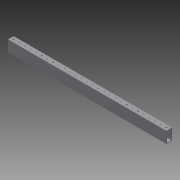
# Autodesk Inventor part: frame_wide
Saved by Autodesk Inventor 2015 SP1 (Build 190203100, 203)
## iProperties
Created: 2014-12-21
Part Number: frame_wide
Material: Generic
Document SubType Name: Modeling
Designer: Jarod
Density: 1 g/cm^3
Appearance: Default
Author: Jarod
Autodesk Inventor part; units mm, degrees
ref_plane "YZ Plane" through (0, 0, 0) normal (1, 0, 0) x (0, 1, 0)
ref_plane "XZ Plane" through (0, 0, 0) normal (0, 1, 0) x (-1, 0, 0)
ref_plane "XY Plane" through (0, 0, 0) normal (0, 0, 1) x (1, 0, 0)
sketch "Sketch1" plane through (0, 0, 0) normal (1, 0, 0) x (0, 1, 0)
  line L0 (0, 0) -> (50.8, 0)
  line L1 (50.8, 0) -> (50.8, -25.4)
  line L2 (50.8, -25.4) -> (0, -25.4)
  line L3 (0, -25.4) -> (0, 0)
  line L4 (2.54, -2.54) -> (48.26, -2.54)
  line L5 (48.26, -2.54) -> (48.26, -22.86)
  line L6 (48.26, -22.86) -> (2.54, -22.86)
  line L7 (2.54, -22.86) -> (2.54, -2.54)
  dimension "d0" = 50.8
  dimension "d1" = 25.4
  dimension "d2" = 45.72
  dimension "d3" = 20.32
  dimension "d4" = 2.54
  dimension "d5" = 2.54
  constraints: 16 end point, 4 parallel, 2 horizontal, 2 perpendicular
  measures "d0" distance of L1.end L2.end
  measures "d1" distance of L0.end L1.end
  measures "d2" distance of L5.end L6.end
  measures "d3" distance of L4.end L5.end
  measures "d4" distance between parallel lines of L4 L0
  measures "d5" distance between parallel lines of L3 L7
extrude "Extrusion1" add sketch "Sketch1" along normal blind 711.2
sketch "Sketch2" plane through (0, 50.8, 0) normal (0, 1, 0) x (1, 0, 0)
  line L0 (0, 0) -> (0, 25.4) projected
  line L1 (0, 0) -> (711.2, 0) projected
  line L2 (711.2, 25.4) -> (711.2, 0) projected
  line L3 (0, 25.4) -> (711.2, 25.4) projected
  line L4 (0, 2.54) -> (0, 22.86) projected
  point P0 (12.7, 12.7)
  dimension "d9" = 12.7
  dimension "d10" = 12.7
  measures "d9" distance from line of point (12.7, 12.7) L0
  measures "d10" distance from line of point (12.7, 12.7) L3
hole "Hole1" at (12.7, 50.8, -12.7) direction (0, -1, 0) diameter 3.9688 end through all
pattern_linear "Rectangular Pattern1" count 28 spacing 25.4 along (1, 0, 0) of "Hole1"
sketch "Sketch4" plane through (0, 50.8, 0) normal (0, 1, 0) x (1, 0, 0)
  circle A0 centre (698.5, 12.7) radius 1.9844 projected
  circle A1 centre (673.1, 12.7) radius 1.9844 projected
  circle A2 centre (647.7, 12.7) radius 1.9844 projected
  circle A3 centre (622.3, 12.7) radius 1.9844 projected
  circle A4 centre (596.9, 12.7) radius 1.9844 projected
  circle A5 centre (571.5, 12.7) radius 1.9844 projected
  circle A6 centre (546.1, 12.7) radius 1.9844 projected
  circle A7 centre (520.7, 12.7) radius 1.9844 projected
  circle A8 centre (495.3, 12.7) radius 1.9844 projected
  circle A9 centre (469.9, 12.7) radius 1.9844 projected
  circle A10 centre (444.5, 12.7) radius 1.9844 projected
  circle A11 centre (419.1, 12.7) radius 1.9844 projected
  circle A12 centre (393.7, 12.7) radius 1.9844 projected
  circle A13 centre (368.3, 12.7) radius 1.9844 projected
  circle A14 centre (342.9, 12.7) radius 1.9844 projected
  circle A15 centre (317.5, 12.7) radius 1.9844 projected
  circle A16 centre (292.1, 12.7) radius 1.9844 projected
  circle A17 centre (266.7, 12.7) radius 1.9844 projected
  circle A18 centre (241.3, 12.7) radius 1.9844 projected
  circle A19 centre (215.9, 12.7) radius 1.9844 projected
  circle A20 centre (190.5, 12.7) radius 1.9844 projected
  circle A21 centre (165.1, 12.7) radius 1.9844 projected
  circle A22 centre (139.7, 12.7) radius 1.9844 projected
  circle A23 centre (114.3, 12.7) radius 1.9844 projected
  circle A24 centre (88.9, 12.7) radius 1.9844 projected
  circle A25 centre (63.5, 12.7) radius 1.9844 projected
  circle A26 centre (38.1, 12.7) radius 1.9844 projected
  circle A27 centre (12.7, 12.7) radius 1.9844 projected
  line L0 (0, 0) -> (0, 25.4) projected
  line L1 (0, 0) -> (711.2, 0) projected
  line L2 (711.2, 25.4) -> (711.2, 0) projected
  line L3 (0, 25.4) -> (711.2, 25.4) projected
  circle A28 centre (12.7, 12.7) radius 1.9844 projected
  circle A29 centre (12.7, 12.7) radius 3.175
  circle A30 centre (139.7, 12.7) radius 3.175
  circle A31 centre (190.5, 12.7) radius 3.175
  circle A32 centre (520.7, 12.7) radius 3.175
  circle A33 centre (571.5, 12.7) radius 1.9844 projected
  circle A34 centre (571.5, 12.7) radius 3.175
  circle A35 centre (698.5, 12.7) radius 1.9844 projected
  circle A36 centre (698.5, 12.7) radius 3.175
  dimension "d27" = 6.35
  dimension "d28" = 6.35
  dimension "d29" = 6.35
  dimension "d30" = 6.35
  dimension "d31" = 6.35
  dimension "d32" = 6.35
  constraints: 6 centre point, 6 coincident
  measures "d27" diameter of A29
  measures "d28" diameter of A30
  measures "d29" diameter of A31
  measures "d30" diameter of A32
  measures "d31" diameter of A34
  measures "d32" diameter of A36
extrude "Extrusion3" cut sketch "Sketch4" against normal blind 25.4 contours A29 | A30 | A31 | A32 | A34 | A36
body "Solid1"
